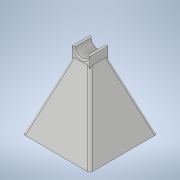
# Autodesk Inventor part: OutdoorSupportForMouseWire
Saved by Autodesk Inventor 2022.1 (Build 261234000, 234)
## iProperties
Created: 2015-07-26
Part Number: OutdoorSupportForMouseWire
Material: Generic
Document SubType Name: Modeling
Designer: steele
Density: 1 g/cm^3
Appearance: Default
Author: steele
Autodesk Inventor part; units mm, degrees
ref_plane "YZ Plane" through (0, 0, 0) normal (1, 0, 0) x (0, 1, 0)
sketch "Sketch1" plane through (0, 0, 0) normal (0, 1, 0) x (-1, 0, 0)
  line L0 (-19.05, 19.05) -> (-19.05, -19.05)
  line L1 (-19.05, -19.05) -> (19.05, -19.05)
  line L2 (19.05, -19.05) -> (19.05, 19.05)
  line L3 (19.05, 19.05) -> (-19.05, 19.05)
  line L4 (-19.05, 19.05) -> (19.05, -19.05) construction
  line L5 (-19.05, -19.05) -> (19.05, 19.05) construction
  point P0 (0, 0)
  dimension "base" = 38.1
  constraints: 12 end point, 2 midpoint, 2 parallel, 2 perpendicular, 1 vertical
  measures "base" distance of L2.end L0.start
ref_plane "Work Plane1" through (0, 38.1, 0) normal (0, 1, 0) x (-1, 0, 0)
sketch "Sketch2" plane through (0, 38.1, 0) normal (0, 1, 0) x (-1, 0, 0)
  line L0 (-5.08, 5.08) -> (-5.08, -5.08)
  line L1 (-5.08, -5.08) -> (5.08, -5.08)
  line L2 (5.08, -5.08) -> (5.08, 5.08)
  line L3 (5.08, 5.08) -> (-5.08, 5.08)
  line L4 (-5.08, 5.08) -> (5.08, -5.08) construction
  line L5 (-5.08, -5.08) -> (5.08, 5.08) construction
  point P0 (0, 0)
  dimension "topOfPyramid" = 10.16
  constraints: 12 end point, 2 midpoint, 2 parallel, 2 perpendicular, 1 vertical
  measures "topOfPyramid" distance of L2.end L0.start
loft "Loft1" add profiles "Sketch1", "Sketch2"
sketch "Sketch3" plane through (0, 0, 0) normal (0, 0, 1) x (1, 0, 0)
  arc A0 (-3.81, 43.18) -> (3.81, 43.18) centre (0, 43.18) ccw
  arc A1 (-5.08, 43.18) -> (5.08, 43.18) centre (0, 43.18) ccw
  line L0 (5.08, 38.1) -> (-5.08, 38.1) projected
  line L1 (3.81, 43.18) -> (5.08, 43.18)
  line L2 (-3.81, 43.18) -> (-5.08, 43.18)
  line L3 (-5.08, 43.18) -> (-5.08, 38.1)
  line L4 (5.08, 43.18) -> (5.08, 38.1)
  line L5 (19.05, 0) -> (5.08, 38.1) projected
  line L6 (5.08, 38.1) -> (0, 38.1)
  line L7 (-5.08, 38.1) -> (5.08, 38.1) projected
  line L8 (-5.08, 38.1) -> (0, 38.1)
  point P0 (0, 0)
  dimension "innerDiamForRope" = 7.62
  dimension "centerForRope" = 5.08
  dimension "outsideDiam" = 10.16
  constraints: 12 end point, 4 point on circle, 2 centre point, 1 coincident, 1 collinear, 1 horizontal, 1 midpoint, 1 perpendicular, 1 point on line, 1 tangent
  measures "innerDiamForRope" diameter of A0
  measures "centerForRope" distance from line of L0 A0.centre
  measures "outsideDiam" diameter of A1
extrude "Extrusion1" add sketch "Sketch3" along normal mid plane 10.16
fillet "Fillet3" radius 1.5875 4 edges at (12.065, 19.05, 12.065) (12.065, 19.05, -12.065) (-12.065, 19.05, 12.065) (-12.065, 19.05, -12.065)
fillet "Fillet5" radius 0.7937 2 edges at (0, 39.37, 5.08) (0, 39.37, -5.08)
ref_plane "Work Plane2" through (0, 0, 19.05) normal (0, 0, 1) x (1, 0, 0)
equation "\"centerForRope\" = 0.5 * outsideDiam"
equation "\"widthOfTop\" = topOfPyramid"
equation "\"d17\" = 0.5 * base"
body "Solid1"
